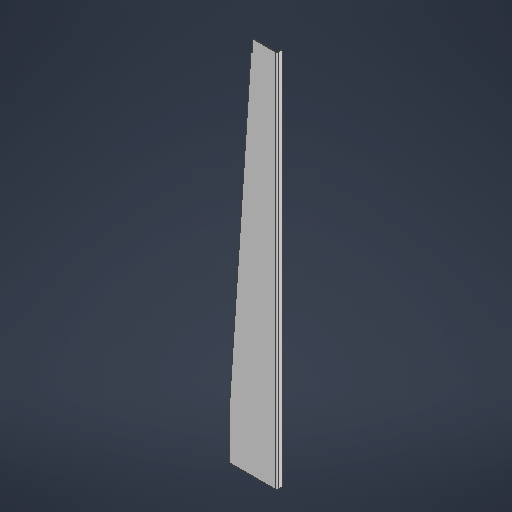
# Autodesk Inventor part: Part2
Saved by Autodesk Inventor 2026.2 (Build 302298000, 298)
## iProperties
Created: 2026-04-17
Part Number: Part2
Material: Generic
Document SubType Name: Sheet Metal
Designer: admin
Density: 1 g/cm^3
Sheet Metal Rule: Default
Appearance: Default
Author: admin
Autodesk Inventor part; units mm, degrees
ref_plane "YZ Plane" through (0, 0, 0) normal (1, 0, 0) x (0, 1, 0)
ref_plane "XZ Plane" through (0, 0, 0) normal (0, 1, 0) x (-1, 0, 0)
ref_plane "XY Plane" through (0, 0, 0) normal (0, 0, 1) x (1, 0, 0)
sketch "Sketch1" plane through (0, 0, 0) normal (0, 0, 1) x (1, 0, 0)
  line L0 (0, 0) -> (0, 1600)
  line L1 (0, 1600) -> (-100, 1600)
  line L2 (-100, 1600) -> (-194.9885, 200)
  line L3 (-194.9885, 200) -> (-194.9885, 0) construction
  line L4 (-194.9885, 0) -> (0, 0)
  line L5 (-103.3847, 1550.1147) -> (-108.3732, 1550.4532)
  line L6 (-108.3732, 1550.4532) -> (-200, 200)
  line L7 (-200, 200) -> (-200, 0)
  line L8 (-200, 0) -> (-194.9885, 0)
  line L9 (-200, 200) -> (-194.9885, 200) construction
  dimension "d0" = 1600
  dimension "d1" = 100
  dimension "d2" = 5
  dimension "d3" = 200
  dimension "d4" = 200
  dimension "d6" = 50
  measures "d0" distance of L0.start L0.end
  measures "d1" distance of L0.end L1.end
  measures "d2" distance of L5.start L5.end
  measures "d3" distance between parallel lines of L0 L7
  measures "d4" distance of L6.end L7.end
  measures "d6" distance from line of L1.end L5
extrude "Plate1" add sketch "Sketch1" along normal blind 3.048
sketch "Sketch2" plane through (-3.048, 0, 3.048) normal (1, 0, 0) x (0, 1, 0)
  line L0 (1600, 0) -> (0, 0)
  line L1 (0, 0) -> (0, -25)
  line L2 (0, -25) -> (1600, -25)
  line L3 (1600, -25) -> (1600, 0)
  constraints: 6 end point, 1 horizontal, 1 perpendicular, 1 vertical
edge flange "Flange1" height 25 angle 90 thickness 3.048 bend radius 3.048 thickness toward (1, 0, 0) relief straight relief width 3.048 relief depth 1.524 edges at (0, 800, 0) wall of the first edge with corners at (-3.048, 1600, 3.048) (-3.048, 0, 3.048) (-3.048, 0, -21.952) (-3.048, 1600, -21.952)
bend "Bend1"
corner "Corner1"
equation "\"d5\" = Thickness"
equation "\"d7\" = BendReliefWidth"
equation "\"d8\" = BendReliefDepth"
equation "\"d9\" = MinimumRemnant"
equation "\"d10\" = TransitionRadius"
equation "\"d13\" = BendRadius"
equation "\"d14\" = CornerReliefSize"
equation "\"d15\" = GapSize"
equation "\"d16\" = JacobiRadiusSize"
equation "\"BendRadius\" = Thickness"
equation "\"BendReliefWidth\" = Thickness"
equation "\"BendReliefDepth\" = 0.5 * Thickness"
equation "\"CornerReliefSize\" = 4 * Thickness"
equation "\"MinimumRemnant\" = 2 * Thickness"
equation "\"TransitionRadius\" = BendRadius"
equation "\"JacobiRadiusSize\" = BendRadius"
equation "\"GapSize\" = Thickness"
equation "\"Thickness\" = 3.048"
body "Solid1"
